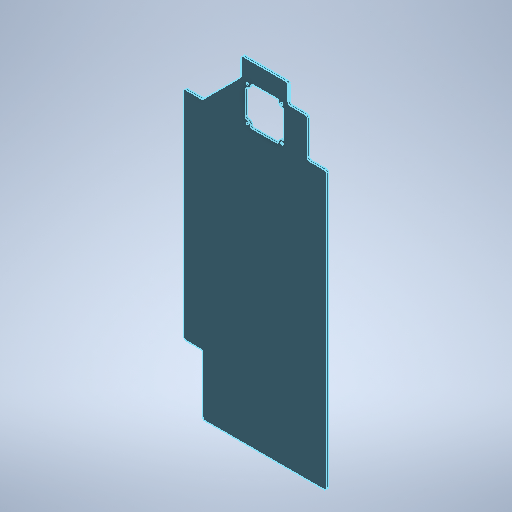
# Autodesk Inventor part: RT_FRM_MC_014_FrontCover_L
Saved by Autodesk Inventor 2025.3 (Build 293356000, 356)
## iProperties
Created: 2026-06-07
Part Number: RT_FRM_MC_014_FrontCover_L
Material: Polycarbonate, Smoke
Document SubType Name: Modeling
Designer: louis
Density: 1.2 g/cm^3
Appearance: Polycarbonate - Smoked
Author: louis
Autodesk Inventor part; units mm, degrees
ref_plane "YZ Plane" through (0, 0, 0) normal (1, 0, 0) x (0, 1, 0)
ref_plane "XZ Plane" through (0, 0, 0) normal (0, 1, 0) x (-1, 0, 0)
ref_plane "XY Plane" through (0, 0, 0) normal (0, 0, 1) x (1, 0, 0)
sketch "Sketch1" plane through (0, 0, 0) normal (0, 0, 1) x (1, 0, 0)
  line L0 (-300, -350) -> (300, -350)
  line L1 (300, -350) -> (300, 350)
  line L2 (300, 350) -> (-300, 350)
  line L3 (-300, 350) -> (-300, -350)
  line L4 (-300, -350) -> (300, 350) construction
  line L5 (300, -350) -> (-300, 350) construction
  line L6 (-80, 310) -> (80, 310)
  line L7 (80, 310) -> (80, 350)
  line L8 (80, 350) -> (-80, 350)
  line L9 (-80, 350) -> (-80, 310)
  line L10 (-80, 310) -> (80, 350) construction
  line L11 (80, 310) -> (-80, 350) construction
  line L12 (-300, 230) -> (-260, 230)
  line L13 (-260, 230) -> (-180, 310)
  line L14 (-180, 310) -> (-180, 350)
  line L15 (180, 350) -> (180, 310)
  line L16 (180, 310) -> (260, 230)
  line L17 (260, 230) -> (300, 230)
  line L18 (-300, -225) -> (-260, -225)
  line L19 (-260, -225) -> (-260, -350)
  line L20 (300, -230) -> (260, -230)
  line L21 (260, -230) -> (260, -350)
  line L22 (0, 0) -> (0, 330) construction
  line L23 (-1, 310) -> (1, 310)
  line L24 (1, 310) -> (1, -350)
  line L25 (1, -350) -> (-1, -350)
  line L26 (-1, -350) -> (-1, 310)
  line L27 (-179, 350) -> (-179, 309.5858)
  line L28 (-179, 309.5858) -> (-259.5858, 229)
  line L29 (-259.5858, 229) -> (-300, 229)
  line L30 (-81, 309) -> (81, 309)
  line L31 (81, 309) -> (81, 351)
  line L32 (81, 351) -> (-81, 351)
  line L33 (-81, 351) -> (-81, 309)
  line L34 (-299, 349) -> (299, 349)
  line L35 (299, 349) -> (299, -349)
  line L36 (299, -349) -> (-299, -349)
  line L37 (-299, -349) -> (-299, 349)
  line L38 (-300, -224) -> (-259, -224)
  line L39 (-259, -224) -> (-259, -350)
  line L40 (259, -350) -> (259, -229)
  line L41 (259, -229) -> (300, -229)
  line L42 (300, 229) -> (259.5858, 229)
  line L43 (259.5858, 229) -> (179, 309.5858)
  line L44 (179, 309.5858) -> (179, 350)
  line L45 (-40, 310) -> (40, 310)
  line L46 (40, 310) -> (40, 230)
  line L47 (40, 230) -> (-40, 230)
  line L48 (-40, 230) -> (-40, 310)
  line L49 (-41, 311) -> (41, 311)
  line L50 (41, 311) -> (41, 229)
  line L51 (41, 229) -> (-41, 229)
  line L52 (-41, 229) -> (-41, 311)
  point P0 (-299, 229)
  point P1 (-299, -224)
  point P2 (-259, -349)
  point P3 (-1, -349)
  point P4 (-1, 309)
  point P5 (-81, 349)
  point P6 (-179, 349)
  point P7 (-1, 229)
  point P8 (-41, 309)
  dimension "d0" = 600
  dimension "d1" = 700
  dimension "d2" = 160
  dimension "d3" = 40
  dimension "d4" = 40
  dimension "d5" = 40
  dimension "d6" = 40
  dimension "d7" = 40
  dimension "d8" = 40
  dimension "d9" = 40
  dimension "d10" = 120
  dimension "d11" = 120
  dimension "d12" = 120
  dimension "d13" = 120
  dimension "d14" = 125
  dimension "d15" = 120
  dimension "d16" = 2
  dimension "d17" = 1
  dimension "d18" = 1
  dimension "d19" = 1
  dimension "d20" = 1
  dimension "d21" = 1
  dimension "d22" = 1
  dimension "d25" = 80
  dimension "d26" = 80
  dimension "d27" = 1
  constraints: 106 end point, 14 parallel, 14 perpendicular, 11 point on line, 5 horizontal, 4 midpoint, 1 collinear, 1 vertical, 17 other
  measures "d0" distance of L2.end L1.end
  measures "d1" distance of L2.end L0.start
  measures "d2" distance of L8.end L7.end
  measures "d3" distance of L7.end L6.end
  measures "d4" distance of L20.start L20.end
  measures "d5" distance of L18.start L18.end
  measures "d6" distance of L12.start L12.end
  measures "d7" distance of L13.end L14.end
  measures "d8" distance of L15.start L15.end
  measures "d9" distance of L16.end L17.end
  measures "d10" distance between parallel lines of L1 L15
  measures "d11" distance between parallel lines of L17 L2
  measures "d12" distance between parallel lines of L2 L12
  measures "d13" distance between parallel lines of L3 L14
  measures "d14" distance of L18.end L19.end
  measures "d15" distance of L20.end L21.end
  measures "d16" distance between parallel lines of L26 L24
  measures "d17" distance between parallel lines of L13 L28
  measures "d18" distance between parallel lines of L9 L33
  measures "d19" distance between parallel lines of L2 L34
  measures "d20" distance between parallel lines of L18 L38
  measures "d21" distance between parallel lines of L21 L40
  measures "d22" distance between parallel lines of L16 L43
  measures "d25" distance of L46.end L47.end
  measures "d26" distance of L45.end L46.end
  measures "d27" distance between parallel lines of L48 L52
extrude "Extrusion1" add sketch "Sketch1" along normal blind 4 contours L39 L38 L37 L29 L28 L27 L34 L33 L30 L52 L51 L26 L36
fillet "Fillet1" radius 4 13 edges at (-179, 349, 2) (-179, 309.5858, 2) (-259.5858, 229, 2) (-299, 229, 2) (-81, 349, 2) (-81, 309, 2) (-41, 309, 2) (-41, 229, 2) (-1, 229, 2) (-1, -349, 2) (-259, -349, 2) (-259, -224, 2) (-299, -224, 2)
sketch "Sketch2" plane through (0, 0, 4) normal (0, 0, 1) x (1, 0, 0)
  arc A0 (-299, -220) -> (-295, -224) centre (-295, -220) ccw projected
  line L0 (-295, -224) -> (-263, -224) projected
  arc A1 (-259, -228) -> (-263, -224) centre (-263, -228) ccw projected
  line L1 (-259, -228) -> (-259, -345) projected
  arc A2 (-259, -345) -> (-255, -349) centre (-255, -345) ccw projected
  line L2 (-255, -349) -> (-5, -349) projected
  arc A3 (-5, -349) -> (-1, -345) centre (-5, -345) ccw projected
  line L3 (-1, -345) -> (-1, 225) projected
  arc A4 (-1, 225) -> (-5, 229) centre (-5, 225) ccw projected
  line L4 (-5, 229) -> (-37, 229) projected
  arc A5 (-41, 233) -> (-37, 229) centre (-37, 233) ccw projected
  line L5 (-41, 233) -> (-41, 305) projected
  arc A6 (-41, 305) -> (-45, 309) centre (-45, 305) ccw projected
  line L6 (-45, 309) -> (-77, 309) projected
  arc A7 (-81, 313) -> (-77, 309) centre (-77, 313) ccw projected
  line L7 (-81, 313) -> (-81, 345) projected
  arc A8 (-81, 345) -> (-85, 349) centre (-85, 345) ccw projected
  line L8 (-85, 349) -> (-175, 349) projected
  arc A9 (-175, 349) -> (-179, 345) centre (-175, 345) ccw projected
  line L9 (-179, 345) -> (-179, 311.2426) projected
  arc A10 (-180.1716, 308.4142) -> (-179, 311.2426) centre (-183, 311.2426) ccw projected
  line L10 (-180.1716, 308.4142) -> (-258.4142, 230.1716) projected
  arc A11 (-261.2426, 229) -> (-258.4142, 230.1716) centre (-261.2426, 233) ccw projected
  line L11 (-261.2426, 229) -> (-295, 229) projected
  arc A12 (-295, 229) -> (-299, 225) centre (-295, 225) ccw projected
  line L12 (-299, 225) -> (-299, -220) projected
  line L13 (-170, 308) -> (-90, 308)
  line L14 (-90, 308) -> (-90, 228)
  line L15 (-90, 228) -> (-170, 228)
  line L16 (-170, 228) -> (-170, 308)
  line L17 (-170, 308) -> (-90, 228) construction
  line L18 (-90, 308) -> (-170, 228) construction
  line L19 (-130, 268) -> (-130, 308) construction
  line L20 (-170, 308) -> (-175, 345) construction
  line L21 (-90, 308) -> (-85, 345) construction
  line L22 (-165.75, 232.25) -> (-94.25, 232.25) construction
  line L23 (-94.25, 232.25) -> (-94.25, 303.75) construction
  line L24 (-94.25, 303.75) -> (-165.75, 303.75) construction
  line L25 (-165.75, 303.75) -> (-165.75, 232.25) construction
  line L26 (-165.75, 232.25) -> (-94.25, 303.75) construction
  line L27 (-94.25, 232.25) -> (-165.75, 303.75) construction
  circle A13 centre (-165.75, 303.75) radius 2.5
  circle A14 centre (-94.25, 303.75) radius 2.5
  circle A15 centre (-94.25, 232.25) radius 2.5
  circle A16 centre (-165.75, 232.25) radius 2.5
  circle A17 centre (-165.75, 303.75) radius 6.5
  line L28 (-165.75, 297.25) -> (-170, 297.25)
  line L29 (-159.25, 303.75) -> (-159.25, 308)
  circle A18 centre (-165.75, 232.25) radius 6.5
  line L30 (-165.75, 238.75) -> (-170, 238.75)
  line L31 (-159.25, 232.25) -> (-159.25, 228)
  circle A19 centre (-94.25, 232.25) radius 6.5
  line L32 (-100.75, 232.25) -> (-100.75, 228)
  line L33 (-94.25, 238.75) -> (-90, 238.75)
  circle A20 centre (-94.25, 303.75) radius 6.5
  line L34 (-94.25, 297.25) -> (-90, 297.25)
  line L35 (-100.75, 303.75) -> (-100.75, 308)
  point P0 (0, 0)
  dimension "d29" = 80
  dimension "d30" = 80
  dimension "d31" = 41
  dimension "d32" = 71.5
  dimension "d33" = 71.5
  dimension "d34" = 5
  dimension "d35" = 5
  dimension "d36" = 5
  dimension "d37" = 5
  dimension "d38" = 4
  dimension "d41" = 360
  constraints: 46 end point, 8 centre point, 8 point on circle, 5 midpoint, 4 coincident, 4 parallel, 4 perpendicular, 4 point on line, 2 horizontal, 2 tangent, 1 equal length, 33 other
  measures "d29" distance of L14.end L15.end
  measures "d30" distance of L13.end L14.end
  measures "d31" distance between parallel lines of L13 L8
  measures "d32" distance of L24.end L23.end
  measures "d33" distance of L22.end L23.end
  measures "d34" diameter of A13
  measures "d35" diameter of A14
  measures "d36" diameter of A15
  measures "d37" diameter of A16
  measures "d38" radial gap between concentric circles of A13 A17
extrude "Extrusion2" cut sketch "Sketch2" against normal blind 4 contours L13 L35 A20 L34 L14 L33 A19 L32 L15 L31 A18 L30 L16 L28 A17 L29 | A13 | A14 | A15 | A16
fillet "Fillet2" radius 4 8 edges at (-100.75, 308, 2) (-90, 297.25, 2) (-90, 238.75, 2) (-100.75, 228, 2) (-159.25, 308, 2) (-170, 297.25, 2) (-170, 238.75, 2) (-159.25, 228, 2)
body "Solid1"
